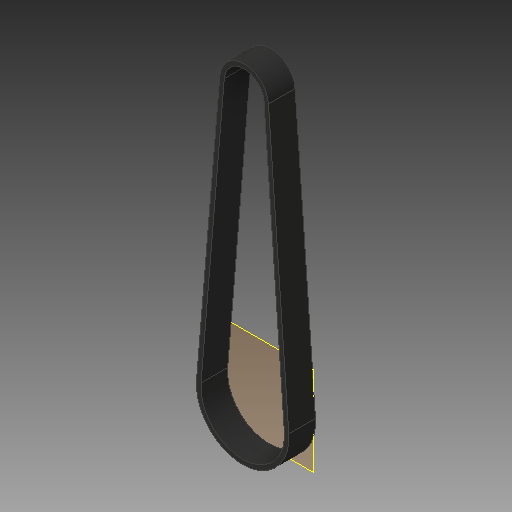
# Autodesk Inventor part: Belt
Saved by Autodesk Inventor 2018.2 (Build 222227000, 227)
## iProperties
Created: 2018-03-28
Part Number: Belt
Material: Rubber
Document SubType Name: Modeling
Designer: Muchen He
Density: 0.93 g/cm^3
Appearance: Rubber - Black
Author: Muchen He
Autodesk Inventor part; units mm, degrees
ref_plane "YZ Plane" through (0, 0, 0) normal (1, 0, 0) x (0, 1, 0)
ref_plane "XZ Plane" through (0, 0, 0) normal (0, 1, 0) x (-1, 0, 0)
ref_plane "Work Plane1" through (0, 0, 1) normal (0, 0, 1) x (1, 0, 0)
sketch "Sketch1" plane through (0, 0, 1) normal (0, 0, 1) x (1, 0, 0)
  circle A0 centre (0, 0) radius 10.7044 projected
  circle A1 centre (0.328, 62.3411) radius 5.7897 projected
  arc A2 (5.8028, 62.7451) -> (-5.1423, 62.8026) centre (0.328, 62.3411) ccw
  arc A3 (-10.3676, 0.8748) -> (10.3762, 0.7656) centre (0, 0) ccw
  line L0 (-5.1423, 62.8026) -> (-10.3676, 0.8748)
  line L1 (5.8028, 62.7451) -> (10.3762, 0.7656)
  arc A4 (-5.1423, 62.8026) -> (5.8028, 62.7451) centre (0.328, 62.3411) ccw construction
  arc A5 (10.3762, 0.7656) -> (-10.3676, 0.8748) centre (0, 0) ccw construction
  line L2 (-9.3711, 0.7907) -> (-4.1458, 62.7186)
  arc A6 (4.8055, 62.6715) -> (-4.1458, 62.7186) centre (0.328, 62.3411) ccw
  line L3 (4.8055, 62.6715) -> (9.3789, 0.6921)
  arc A7 (-9.3711, 0.7907) -> (9.3789, 0.6921) centre (0, 0) ccw
  point P0 (0, 0)
  dimension "d1" = 0.3
  dimension "d2" = 0.3
  dimension "d3" = 1
  constraints: 12 point on circle, 8 end point, 6 centre point, 4 tangent, 3 other
  measures "d1" radial gap between concentric circles of A1 A2
  measures "d2" radial gap between concentric circles of A0 A3
  measures "d3" distance between parallel lines of L0 L2
extrude "Extrusion1" add sketch "Sketch1" along normal blind 6 contours L1 A3 L0 A0 L2 A7 L3 | A0 L3 A1 L1 | L0 A1 L2 A0 | A1 L3 A6 L2 L0 A2 L1
body "Solid1"
